Autodesk Fusion 360 part; units mm, degrees
(part 4 of 5)
  line L171 (98.6977, -61.525) -> (108.6977, -61.525)
  arc A178 (108.6977, -84.525) -> (108.6977, -81.525) centre (108.6977, -83.025) ccw
  line L172 (108.6977, -84.525) -> (98.6977, -84.525)
  arc A179 (98.6977, -81.525) -> (98.6977, -84.525) centre (98.6977, -83.025) ccw
  line L173 (98.6977, -81.525) -> (108.6977, -81.525)
  arc A180 (228.6977, -154.525) -> (228.6977, -151.525) centre (228.6977, -153.025) ccw
  line L174 (228.6977, -154.525) -> (218.6977, -154.525)
  arc A181 (218.6977, -151.525) -> (218.6977, -154.525) centre (218.6977, -153.025) ccw
  line L175 (218.6977, -151.525) -> (228.6977, -151.525)
  arc A182 (188.6977, -154.525) -> (188.6977, -151.525) centre (188.6977, -153.025) ccw
  line L176 (188.6977, -154.525) -> (178.6977, -154.525)
  arc A183 (178.6977, -151.525) -> (178.6977, -154.525) centre (178.6977, -153.025) ccw
  line L177 (178.6977, -151.525) -> (188.6977, -151.525)
  arc A184 (108.6977, -74.525) -> (108.6977, -71.525) centre (108.6977, -73.025) ccw
  line L178 (108.6977, -74.525) -> (98.6977, -74.525)
  arc A185 (98.6977, -71.525) -> (98.6977, -74.525) centre (98.6977, -73.025) ccw
  line L179 (98.6977, -71.525) -> (108.6977, -71.525)
  arc A186 (88.6977, -64.525) -> (88.6977, -61.525) centre (88.6977, -63.025) ccw
  line L180 (88.6977, -64.525) -> (78.6977, -64.525)
  arc A187 (78.6977, -61.525) -> (78.6977, -64.525) centre (78.6977, -63.025) ccw
  line L181 (78.6977, -61.525) -> (88.6977, -61.525)
  arc A188 (168.6977, -114.525) -> (168.6977, -111.525) centre (168.6977, -113.025) ccw
  line L182 (168.6977, -114.525) -> (158.6977, -114.525)
  arc A189 (158.6977, -111.525) -> (158.6977, -114.525) centre (158.6977, -113.025) ccw
  line L183 (158.6977, -111.525) -> (168.6977, -111.525)
  arc A190 (228.6977, -94.525) -> (228.6977, -91.525) centre (228.6977, -93.025) ccw
  line L184 (228.6977, -94.525) -> (218.6977, -94.525)
  arc A191 (218.6977, -91.525) -> (218.6977, -94.525) centre (218.6977, -93.025) ccw
  line L185 (218.6977, -91.525) -> (228.6977, -91.525)
  arc A192 (208.6977, -84.525) -> (208.6977, -81.525) centre (208.6977, -83.025) ccw
  line L186 (208.6977, -84.525) -> (198.6977, -84.525)
  arc A193 (198.6977, -81.525) -> (198.6977, -84.525) centre (198.6977, -83.025) ccw
  line L187 (198.6977, -81.525) -> (208.6977, -81.525)
  arc A194 (88.6977, -54.525) -> (88.6977, -51.525) centre (88.6977, -53.025) ccw
  line L188 (88.6977, -54.525) -> (78.6977, -54.525)
  arc A195 (78.6977, -51.525) -> (78.6977, -54.525) centre (78.6977, -53.025) ccw
  line L189 (78.6977, -51.525) -> (88.6977, -51.525)
  arc A196 (188.6977, -14.525) -> (188.6977, -11.525) centre (188.6977, -13.025) ccw
  line L190 (188.6977, -14.525) -> (178.6977, -14.525)
  arc A197 (178.6977, -11.525) -> (178.6977, -14.525) centre (178.6977, -13.025) ccw
  line L191 (178.6977, -11.525) -> (188.6977, -11.525)
  arc A198 (148.6977, -184.525) -> (148.6977, -181.525) centre (148.6977, -183.025) ccw
  line L192 (148.6977, -184.525) -> (138.6977, -184.525)
  arc A199 (138.6977, -181.525) -> (138.6977, -184.525) centre (138.6977, -183.025) ccw
  line L193 (138.6977, -181.525) -> (148.6977, -181.525)
  arc A200 (208.6977, -54.525) -> (208.6977, -51.525) centre (208.6977, -53.025) ccw
  line L194 (208.6977, -54.525) -> (198.6977, -54.525)
  arc A201 (198.6977, -51.525) -> (198.6977, -54.525) centre (198.6977, -53.025) ccw
  line L195 (198.6977, -51.525) -> (208.6977, -51.525)
  arc A202 (68.6977, -54.525) -> (68.6977, -51.525) centre (68.6977, -53.025) ccw
  line L196 (68.6977, -54.525) -> (58.6977, -54.525)
  arc A203 (58.6977, -51.525) -> (58.6977, -54.525) centre (58.6977, -53.025) ccw
  line L197 (58.6977, -51.525) -> (68.6977, -51.525)
  arc A204 (208.6977, -64.525) -> (208.6977, -61.525) centre (208.6977, -63.025) ccw
  line L198 (208.6977, -64.525) -> (198.6977, -64.525)
  arc A205 (198.6977, -61.525) -> (198.6977, -64.525) centre (198.6977, -63.025) ccw
  line L199 (198.6977, -61.525) -> (208.6977, -61.525)
  arc A206 (208.6977, -174.525) -> (208.6977, -171.525) centre (208.6977, -173.025) ccw
  line L200 (208.6977, -174.525) -> (198.6977, -174.525)
  arc A207 (198.6977, -171.525) -> (198.6977, -174.525) centre (198.6977, -173.025) ccw
  line L201 (198.6977, -171.525) -> (208.6977, -171.525)
  arc A208 (168.6977, -144.525) -> (168.6977, -141.525) centre (168.6977, -143.025) ccw
  line L202 (168.6977, -144.525) -> (158.6977, -144.525)
  arc A209 (158.6977, -141.525) -> (158.6977, -144.525) centre (158.6977, -143.025) ccw
  line L203 (158.6977, -141.525) -> (168.6977, -141.525)
  arc A210 (68.6977, -64.525) -> (68.6977, -61.525) centre (68.6977, -63.025) ccw
  line L204 (68.6977, -64.525) -> (58.6977, -64.525)
  arc A211 (58.6977, -61.525) -> (58.6977, -64.525) centre (58.6977, -63.025) ccw
  line L205 (58.6977, -61.525) -> (68.6977, -61.525)
  arc A212 (248.6977, -124.525) -> (248.6977, -121.525) centre (248.6977, -123.025) ccw
  line L206 (248.6977, -124.525) -> (238.6977, -124.525)
  arc A213 (238.6977, -121.525) -> (238.6977, -124.525) centre (238.6977, -123.025) ccw
  line L207 (238.6977, -121.525) -> (248.6977, -121.525)
  arc A214 (228.6977, -124.525) -> (228.6977, -121.525) centre (228.6977, -123.025) ccw
  line L208 (228.6977, -124.525) -> (218.6977, -124.525)
  arc A215 (218.6977, -121.525) -> (218.6977, -124.525) centre (218.6977, -123.025) ccw
  line L209 (218.6977, -121.525) -> (228.6977, -121.525)
  arc A216 (208.6977, -144.525) -> (208.6977, -141.525) centre (208.6977, -143.025) ccw
  line L210 (208.6977, -144.525) -> (198.6977, -144.525)
  arc A217 (198.6977, -141.525) -> (198.6977, -144.525) centre (198.6977, -143.025) ccw
  line L211 (198.6977, -141.525) -> (208.6977, -141.525)
  arc A218 (148.6977, -134.525) -> (148.6977, -131.525) centre (148.6977, -133.025) ccw
  line L212 (148.6977, -134.525) -> (138.6977, -134.525)
  arc A219 (138.6977, -131.525) -> (138.6977, -134.525) centre (138.6977, -133.025) ccw
  line L213 (138.6977, -131.525) -> (148.6977, -131.525)
  arc A220 (188.6977, -64.525) -> (188.6977, -61.525) centre (188.6977, -63.025) ccw
  line L214 (188.6977, -64.525) -> (178.6977, -64.525)
  arc A221 (178.6977, -61.525) -> (178.6977, -64.525) centre (178.6977, -63.025) ccw
  line L215 (178.6977, -61.525) -> (188.6977, -61.525)
  arc A222 (168.6977, -174.525) -> (168.6977, -171.525) centre (168.6977, -173.025) ccw
  line L216 (168.6977, -174.525) -> (158.6977, -174.525)
  arc A223 (158.6977, -171.525) -> (158.6977, -174.525) centre (158.6977, -173.025) ccw
  line L217 (158.6977, -171.525) -> (168.6977, -171.525)
  arc A224 (228.6977, -114.525) -> (228.6977, -111.525) centre (228.6977, -113.025) ccw
  line L218 (228.6977, -114.525) -> (218.6977, -114.525)
  arc A225 (218.6977, -111.525) -> (218.6977, -114.525) centre (218.6977, -113.025) ccw
  line L219 (218.6977, -111.525) -> (228.6977, -111.525)
  arc A226 (128.6977, -94.525) -> (128.6977, -91.525) centre (128.6977, -93.025) ccw
  line L220 (128.6977, -94.525) -> (118.6977, -94.525)
  arc A227 (118.6977, -91.525) -> (118.6977, -94.525) centre (118.6977, -93.025) ccw
  line L221 (118.6977, -91.525) -> (128.6977, -91.525)
  arc A228 (168.6977, 5.475) -> (168.6977, 8.475) centre (168.6977, 6.975) ccw
  line L222 (168.6977, 5.475) -> (158.6977, 5.475)
  arc A229 (158.6977, 8.475) -> (158.6977, 5.475) centre (158.6977, 6.975) ccw
  line L223 (158.6977, 8.475) -> (168.6977, 8.475)
  arc A230 (188.6977, -74.525) -> (188.6977, -71.525) centre (188.6977, -73.025) ccw
  line L224 (188.6977, -74.525) -> (178.6977, -74.525)
  arc A231 (178.6977, -71.525) -> (178.6977, -74.525) centre (178.6977, -73.025) ccw
  line L225 (178.6977, -71.525) -> (188.6977, -71.525)
  arc A232 (108.6977, -114.525) -> (108.6977, -111.525) centre (108.6977, -113.025) ccw
  line L226 (108.6977, -114.525) -> (98.6977, -114.525)
  arc A233 (98.6977, -111.525) -> (98.6977, -114.525) centre (98.6977, -113.025) ccw
  line L227 (98.6977, -111.525) -> (108.6977, -111.525)
  arc A234 (208.6977, -104.525) -> (208.6977, -101.525) centre (208.6977, -103.025) ccw
  line L228 (208.6977, -104.525) -> (198.6977, -104.525)
  arc A235 (198.6977, -101.525) -> (198.6977, -104.525) centre (198.6977, -103.025) ccw
  line L229 (198.6977, -101.525) -> (208.6977, -101.525)
  arc A236 (208.6977, -154.525) -> (208.6977, -151.525) centre (208.6977, -153.025) ccw
  line L230 (208.6977, -154.525) -> (198.6977, -154.525)
  arc A237 (198.6977, -151.525) -> (198.6977, -154.525) centre (198.6977, -153.025) ccw
  line L231 (198.6977, -151.525) -> (208.6977, -151.525)
  arc A238 (168.6977, -104.525) -> (168.6977, -101.525) centre (168.6977, -103.025) ccw
  line L232 (168.6977, -104.525) -> (158.6977, -104.525)
  arc A239 (158.6977, -101.525) -> (158.6977, -104.525) centre (158.6977, -103.025) ccw
  line L233 (158.6977, -101.525) -> (168.6977, -101.525)
  arc A240 (188.6977, -174.525) -> (188.6977, -171.525) centre (188.6977, -173.025) ccw
  line L234 (188.6977, -174.525) -> (178.6977, -174.525)
  arc A241 (178.6977, -171.525) -> (178.6977, -174.525) centre (178.6977, -173.025) ccw
  line L235 (178.6977, -171.525) -> (188.6977, -171.525)
  arc A242 (248.6977, -64.525) -> (248.6977, -61.525) centre (248.6977, -63.025) ccw
  line L236 (248.6977, -64.525) -> (238.6977, -64.525)
  arc A243 (238.6977, -61.525) -> (238.6977, -64.525) centre (238.6977, -63.025) ccw
  line L237 (238.6977, -61.525) -> (248.6977, -61.525)
  arc A244 (128.6977, -84.525) -> (128.6977, -81.525) centre (128.6977, -83.025) ccw
  line L238 (128.6977, -84.525) -> (118.6977, -84.525)
  arc A245 (118.6977, -81.525) -> (118.6977, -84.525) centre (118.6977, -83.025) ccw
  line L239 (118.6977, -81.525) -> (128.6977, -81.525)
  arc A246 (88.6977, -114.525) -> (88.6977, -111.525) centre (88.6977, -113.025) ccw
  line L240 (88.6977, -114.525) -> (78.6977, -114.525)
  arc A247 (78.6977, -111.525) -> (78.6977, -114.525) centre (78.6977, -113.025) ccw
  line L241 (78.6977, -111.525) -> (88.6977, -111.525)
  line L242 (46.3999, -83.0262) -> (46.3999, -63.0262)
  line L243 (46.3999, -63.0262) -> (53.3999, -63.0262)
  line L244 (53.3999, -63.0262) -> (53.3999, -83.0262)
  line L245 (53.3999, -83.0262) -> (46.3999, -83.0262)
  arc A248 (230.0109, -143.75) -> (228.6869, -141.525) centre (230, -142.25) ccw
  arc A249 (228.6977, -144.525) -> (230.0109, -143.75) centre (228.6977, -143.025) ccw
  line L246 (228.6977, -144.525) -> (218.6977, -144.525)
  arc A250 (218.6977, -141.525) -> (218.6977, -144.525) centre (218.6977, -143.025) ccw
  line L247 (218.6977, -141.525) -> (228.6869, -141.525)
  arc A251 (168.6977, -94.525) -> (168.6977, -91.525) centre (168.6977, -93.025) ccw
  line L248 (168.6977, -94.525) -> (158.6977, -94.525)
  arc A252 (158.6977, -91.525) -> (158.6977, -94.525) centre (158.6977, -93.025) ccw
  line L249 (158.6977, -91.525) -> (168.6977, -91.525)
  arc A253 (248.6977, -114.525) -> (248.6977, -111.525) centre (248.6977, -113.025) ccw
  line L250 (248.6977, -114.525) -> (238.6977, -114.525)
  arc A254 (238.6977, -111.525) -> (238.6977, -114.525) centre (238.6977, -113.025) ccw
  line L251 (238.6977, -111.525) -> (248.6977, -111.525)
  arc A255 (168.6977, -54.525) -> (168.6977, -51.525) centre (168.6977, -53.025) ccw
  line L252 (168.6977, -54.525) -> (158.6977, -54.525)
  arc A256 (158.6977, -51.525) -> (158.6977, -54.525) centre (158.6977, -53.025) ccw
  line L253 (158.6977, -51.525) -> (168.6977, -51.525)
  arc A257 (168.6977, -74.525) -> (168.6977, -71.525) centre (168.6977, -73.025) ccw
  line L254 (168.6977, -74.525) -> (158.6977, -74.525)
  arc A258 (158.6977, -71.525) -> (158.6977, -74.525) centre (158.6977, -73.025) ccw
  line L255 (158.6977, -71.525) -> (168.6977, -71.525)
  arc A259 (248.6977, -104.525) -> (248.6977, -101.525) centre (248.6977, -103.025) ccw
  line L256 (248.6977, -104.525) -> (238.6977, -104.525)
  arc A260 (238.6977, -101.525) -> (238.6977, -104.525) centre (238.6977, -103.025) ccw
  line L257 (238.6977, -101.525) -> (248.6977, -101.525)
  arc A261 (228.6977, -164.525) -> (228.6977, -161.525) centre (228.6977, -163.025) ccw
  line L258 (228.6977, -164.525) -> (218.6977, -164.525)
  arc A262 (218.6977, -161.525) -> (218.6977, -164.525) centre (218.6977, -163.025) ccw
  line L259 (218.6977, -161.525) -> (228.6977, -161.525)
  arc A263 (208.6977, -164.525) -> (208.6977, -161.525) centre (208.6977, -163.025) ccw
  line L260 (208.6977, -164.525) -> (198.6977, -164.525)
  arc A264 (198.6977, -161.525) -> (198.6977, -164.525) centre (198.6977, -163.025) ccw
  line L261 (198.6977, -161.525) -> (208.6977, -161.525)
  arc A265 (188.6977, -144.525) -> (188.6977, -141.525) centre (188.6977, -143.025) ccw
  line L262 (188.6977, -144.525) -> (178.6977, -144.525)
  arc A266 (178.6977, -141.525) -> (178.6977, -144.525) centre (178.6977, -143.025) ccw
  line L263 (178.6977, -141.525) -> (188.6977, -141.525)
  arc A267 (188.6977, 35.475) -> (188.6977, 38.475) centre (188.6977, 36.975) ccw
  line L264 (188.6977, 35.475) -> (178.6977, 35.475)
  arc A268 (178.6977, 38.475) -> (178.6977, 35.475) centre (178.6977, 36.975) ccw
  line L265 (178.6977, 38.475) -> (188.6977, 38.475)
  arc A269 (188.6977, -54.525) -> (188.6977, -51.525) centre (188.6977, -53.025) ccw
  line L266 (188.6977, -54.525) -> (178.6977, -54.525)
  arc A270 (178.6977, -51.525) -> (178.6977, -54.525) centre (178.6977, -53.025) ccw
  line L267 (178.6977, -51.525) -> (188.6977, -51.525)
  arc A271 (128.6977, -134.525) -> (128.6977, -131.525) centre (128.6977, -133.025) ccw
  line L268 (128.6977, -134.525) -> (118.6977, -134.525)
  arc A272 (118.6977, -131.525) -> (118.6977, -134.525) centre (118.6977, -133.025) ccw
  line L269 (118.6977, -131.525) -> (128.6977, -131.525)
  arc A273 (88.6977, -84.525) -> (88.6977, -81.525) centre (88.6977, -83.025) ccw
  line L270 (88.6977, -84.525) -> (78.6977, -84.525)
  arc A274 (78.6977, -81.525) -> (78.6977, -84.525) centre (78.6977, -83.025) ccw
  line L271 (78.6977, -81.525) -> (88.6977, -81.525)
  arc A275 (188.6977, -84.525) -> (188.6977, -81.525) centre (188.6977, -83.025) ccw
  line L272 (188.6977, -84.525) -> (178.6977, -84.525)
  arc A276 (178.6977, -81.525) -> (178.6977, -84.525) centre (178.6977, -83.025) ccw
  line L273 (178.6977, -81.525) -> (188.6977, -81.525)
  arc A277 (188.6977, 15.475) -> (188.6977, 18.475) centre (188.6977, 16.975) ccw
  line L274 (188.6977, 15.475) -> (178.6977, 15.475)
  arc A278 (178.6977, 18.475) -> (178.6977, 15.475) centre (178.6977, 16.975) ccw
  line L275 (178.6977, 18.475) -> (188.6977, 18.475)
  arc A279 (128.6977, -114.525) -> (128.6977, -111.525) centre (128.6977, -113.025) ccw
  line L276 (128.6977, -114.525) -> (118.6977, -114.525)
  arc A280 (118.6977, -111.525) -> (118.6977, -114.525) centre (118.6977, -113.025) ccw
  line L277 (118.6977, -111.525) -> (128.6977, -111.525)
  arc A281 (248.6977, -84.525) -> (248.6977, -81.525) centre (248.6977, -83.025) ccw
  line L278 (248.6977, -84.525) -> (238.6977, -84.525)
  arc A282 (238.6977, -81.525) -> (238.6977, -84.525) centre (238.6977, -83.025) ccw
  line L279 (238.6977, -81.525) -> (248.6977, -81.525)
  arc A283 (88.6977, -104.525) -> (88.6977, -101.525) centre (88.6977, -103.025) ccw
  line L280 (88.6977, -104.525) -> (78.6977, -104.525)
  arc A284 (78.6977, -101.525) -> (78.6977, -104.525) centre (78.6977, -103.025) ccw
  line L281 (78.6977, -101.525) -> (88.6977, -101.525)
  arc A285 (128.6977, -154.525) -> (128.6977, -151.525) centre (128.6977, -153.025) ccw
  line L282 (128.6977, -154.525) -> (118.6977, -154.525)
  arc A286 (118.6977, -151.525) -> (118.6977, -154.525) centre (118.6977, -153.025) ccw
  line L283 (118.6977, -151.525) -> (128.6977, -151.525)
  arc A287 (228.6977, -104.525) -> (228.6977, -101.525) centre (228.6977, -103.025) ccw
  line L284 (228.6977, -104.525) -> (218.6977, -104.525)
  arc A288 (218.6977, -101.525) -> (218.6977, -104.525) centre (218.6977, -103.025) ccw
  line L285 (218.6977, -101.525) -> (228.6977, -101.525)
  arc A289 (188.6977, -134.525) -> (188.6977, -131.525) centre (188.6977, -133.025) ccw
  line L286 (188.6977, -134.525) -> (178.6977, -134.525)
  arc A290 (178.6977, -131.525) -> (178.6977, -134.525) centre (178.6977, -133.025) ccw
  line L287 (178.6977, -131.525) -> (188.6977, -131.525)
  arc A291 (228.6977, -74.525) -> (228.6977, -71.525) centre (228.6977, -73.025) ccw
  line L288 (228.6977, -74.525) -> (218.6977, -74.525)
  arc A292 (218.6977, -71.525) -> (218.6977, -74.525) centre (218.6977, -73.025) ccw
  line L289 (218.6977, -71.525) -> (228.6977, -71.525)
  arc A293 (188.6977, -104.525) -> (188.6977, -101.525) centre (188.6977, -103.025) ccw
  line L290 (188.6977, -104.525) -> (178.6977, -104.525)
  arc A294 (178.6977, -101.525) -> (178.6977, -104.525) centre (178.6977, -103.025) ccw
  line L291 (178.6977, -101.525) -> (188.6977, -101.525)
  arc A295 (208.6977, -124.525) -> (208.6977, -121.525) centre (208.6977, -123.025) ccw
  line L292 (208.6977, -124.525) -> (198.6977, -124.525)
  arc A296 (198.6977, -121.525) -> (198.6977, -124.525) centre (198.6977, -123.025) ccw
  line L293 (198.6977, -121.525) -> (208.6977, -121.525)
  arc A297 (68.6977, -84.525) -> (68.6977, -81.525) centre (68.6977, -83.025) ccw
  line L294 (68.6977, -84.525) -> (58.6977, -84.525)
  arc A298 (58.6977, -81.525) -> (58.6977, -84.525) centre (58.6977, -83.025) ccw
  line L295 (58.6977, -81.525) -> (68.6977, -81.525)
  arc A299 (148.6977, -54.525) -> (148.6977, -51.525) centre (148.6977, -53.025) ccw
  line L296 (148.6977, -54.525) -> (138.6977, -54.525)
  arc A300 (138.6977, -51.525) -> (138.6977, -54.525) centre (138.6977, -53.025) ccw
  line L297 (138.6977, -51.525) -> (148.6977, -51.525)
  arc A301 (248.6977, -94.525) -> (248.6977, -91.525) centre (248.6977, -93.025) ccw
  line L298 (248.6977, -94.525) -> (238.6977, -94.525)
  arc A302 (238.6977, -91.525) -> (238.6977, -94.525) centre (238.6977, -93.025) ccw
  line L299 (238.6977, -91.525) -> (248.6977, -91.525)
  arc A303 (208.6977, -184.525) -> (208.6977, -181.525) centre (208.6977, -183.025) ccw
  line L300 (208.6977, -184.525) -> (198.6977, -184.525)
  arc A304 (198.6977, -181.525) -> (198.6977, -184.525) centre (198.6977, -183.025) ccw
  line L301 (198.6977, -181.525) -> (208.6977, -181.525)
  arc A305 (108.6977, -94.525) -> (108.6977, -91.525) centre (108.6977, -93.025) ccw
  line L302 (108.6977, -94.525) -> (98.6977, -94.525)
  arc A306 (98.6977, -91.525) -> (98.6977, -94.525) centre (98.6977, -93.025) ccw
  line L303 (98.6977, -91.525) -> (108.6977, -91.525)
  arc A307 (128.6977, -14.525) -> (128.6977, -11.525) centre (128.6977, -13.025) ccw
  line L304 (128.6977, -14.525) -> (118.6977, -14.525)
  arc A308 (118.6977, -11.525) -> (118.6977, -14.525) centre (118.6977, -13.025) ccw
  line L305 (118.6977, -11.525) -> (128.6977, -11.525)
  arc A309 (188.6977, -94.525) -> (188.6977, -91.525) centre (188.6977, -93.025) ccw
  line L306 (188.6977, -94.525) -> (178.6977, -94.525)
  arc A310 (178.6977, -91.525) -> (178.6977, -94.525) centre (178.6977, -93.025) ccw
  line L307 (178.6977, -91.525) -> (188.6977, -91.525)
  arc A311 (168.6977, -134.525) -> (168.6977, -131.525) centre (168.6977, -133.025) ccw
  line L308 (168.6977, -134.525) -> (158.6977, -134.525)
  arc A312 (158.6977, -131.525) -> (158.6977, -134.525) centre (158.6977, -133.025) ccw
  line L309 (158.6977, -131.525) -> (168.6977, -131.525)
  arc A313 (128.6977, -144.525) -> (128.6977, -141.525) centre (128.6977, -143.025) ccw
  line L310 (128.6977, -144.525) -> (118.6977, -144.525)
  arc A314 (118.6977, -141.525) -> (118.6977, -144.525) centre (118.6977, -143.025) ccw
  line L311 (118.6977, -141.525) -> (128.6977, -141.525)
  arc A315 (88.6977, -74.525) -> (88.6977, -71.525) centre (88.6977, -73.025) ccw
  line L312 (88.6977, -74.525) -> (78.6977, -74.525)
  arc A316 (78.6977, -71.525) -> (78.6977, -74.525) centre (78.6977, -73.025) ccw
  line L313 (78.6977, -71.525) -> (88.6977, -71.525)
  arc A317 (148.6977, -84.525) -> (148.6977, -81.525) centre (148.6977, -83.025) ccw
  line L314 (148.6977, -84.525) -> (138.6977, -84.525)
  arc A318 (138.6977, -81.525) -> (138.6977, -84.525) centre (138.6977, -83.025) ccw
  line L315 (138.6977, -81.525) -> (148.6977, -81.525)
  arc A319 (108.6977, -104.525) -> (108.6977, -101.525) centre (108.6977, -103.025) ccw
  line L316 (108.6977, -104.525) -> (98.6977, -104.525)
  arc A320 (98.6977, -101.525) -> (98.6977, -104.525) centre (98.6977, -103.025) ccw
  line L317 (98.6977, -101.525) -> (108.6977, -101.525)
  arc A321 (168.6977, -84.525) -> (168.6977, -81.525) centre (168.6977, -83.025) ccw
  line L318 (168.6977, -84.525) -> (158.6977, -84.525)
  arc A322 (158.6977, -81.525) -> (158.6977, -84.525) centre (158.6977, -83.025) ccw
  line L319 (158.6977, -81.525) -> (168.6977, -81.525)
  arc A323 (228.6977, -64.525) -> (228.6977, -61.525) centre (228.6977, -63.025) ccw
  line L320 (228.6977, -64.525) -> (218.6977, -64.525)
  arc A324 (218.6977, -61.525) -> (218.6977, -64.525) centre (218.6977, -63.025) ccw
  line L321 (218.6977, -61.525) -> (228.6977, -61.525)
  arc A325 (228.6977, -84.525) -> (228.6977, -81.525) centre (228.6977, -83.025) ccw
  line L322 (228.6977, -84.525) -> (218.6977, -84.525)
  arc A326 (218.6977, -81.525) -> (218.6977, -84.525) centre (218.6977, -83.025) ccw
  line L323 (218.6977, -81.525) -> (228.6977, -81.525)
  arc A327 (148.6977, -114.525) -> (148.6977, -111.525) centre (148.6977, -113.025) ccw
  line L324 (148.6977, -114.525) -> (138.6977, -114.525)
  arc A328 (138.6977, -111.525) -> (138.6977, -114.525) centre (138.6977, -113.025) ccw
  line L325 (138.6977, -111.525) -> (148.6977, -111.525)
  arc A329 (168.6977, -154.525) -> (168.6977, -151.525) centre (168.6977, -153.025) ccw
  line L326 (168.6977, -154.525) -> (158.6977, -154.525)
  arc A330 (158.6977, -151.525) -> (158.6977, -154.525) centre (158.6977, -153.025) ccw
  line L327 (158.6977, -151.525) -> (168.6977, -151.525)
  arc A331 (68.6977, -74.525) -> (68.6977, -71.525) centre (68.6977, -73.025) ccw
  line L328 (68.6977, -74.525) -> (58.6977, -74.525)
  arc A332 (58.6977, -71.525) -> (58.6977, -74.525) centre (58.6977, -73.025) ccw
  line L329 (58.6977, -71.525) -> (68.6977, -71.525)
  arc A333 (128.6977, -64.525) -> (128.6977, -61.525) centre (128.6977, -63.025) ccw
  line L330 (128.6977, -64.525) -> (118.6977, -64.525)
  arc A334 (118.6977, -61.525) -> (118.6977, -64.525) centre (118.6977, -63.025) ccw
  line L331 (118.6977, -61.525) -> (128.6977, -61.525)
  arc A335 (248.6977, -134.525) -> (248.6977, -131.525) centre (248.6977, -133.025) ccw
  line L332 (248.6977, -134.525) -> (238.6977, -134.525)
  arc A336 (238.6977, -131.525) -> (238.6977, -134.525) centre (238.6977, -133.025) ccw
  line L333 (238.6977, -131.525) -> (248.6977, -131.525)
  arc A337 (128.6977, -104.525) -> (128.6977, -101.525) centre (128.6977, -103.025) ccw
  line L334 (128.6977, -104.525) -> (118.6977, -104.525)
  arc A338 (118.6977, -101.525) -> (118.6977, -104.525) centre (118.6977, -103.025) ccw
  line L335 (118.6977, -101.525) -> (128.6977, -101.525)
  arc A339 (208.6977, -4.525) -> (208.6977, -1.525) centre (208.6977, -3.025) ccw
  line L336 (208.6977, -4.525) -> (198.6977, -4.525)
  arc A340 (198.6977, -1.525) -> (198.6977, -4.525) centre (198.6977, -3.025) ccw
  line L337 (198.6977, -1.525) -> (208.6977, -1.525)
  arc A341 (208.6977, -134.525) -> (208.6977, -131.525) centre (208.6977, -133.025) ccw
  line L338 (208.6977, -134.525) -> (198.6977, -134.525)
  arc A342 (198.6977, -131.525) -> (198.6977, -134.525) centre (198.6977, -133.025) ccw
  line L339 (198.6977, -131.525) -> (208.6977, -131.525)
  arc A343 (128.6977, -124.525) -> (128.6977, -121.525) centre (128.6977, -123.025) ccw
  line L340 (128.6977, -124.525) -> (118.6977, -124.525)
  arc A344 (118.6977, -121.525) -> (118.6977, -124.525) centre (118.6977, -123.025) ccw
  line L341 (118.6977, -121.525) -> (128.6977, -121.525)
  arc A345 (128.6977, -54.525) -> (128.6977, -51.525) centre (128.6977, -53.025) ccw
  line L342 (128.6977, -54.525) -> (118.6977, -54.525)
  arc A346 (118.6977, -51.525) -> (118.6977, -54.525) centre (118.6977, -53.025) ccw
  line L343 (118.6977, -51.525) -> (128.6977, -51.525)
  arc A347 (208.6977, -14.525) -> (208.6977, -11.525) centre (208.6977, -13.025) ccw
  line L344 (208.6977, -14.525) -> (198.6977, -14.525)
  arc A348 (198.6977, -11.525) -> (198.6977, -14.525) centre (198.6977, -13.025) ccw
  line L345 (198.6977, -11.525) -> (208.6977, -11.525)
  arc A349 (108.6977, -134.525) -> (108.6977, -131.525) centre (108.6977, -133.025) ccw
  line L346 (108.6977, -134.525) -> (98.6977, -134.525)
  arc A350 (98.6977, -131.525) -> (98.6977, -134.525) centre (98.6977, -133.025) ccw
  line L347 (98.6977, -131.525) -> (108.6977, -131.525)
  arc A351 (88.6977, -94.525) -> (88.6977, -91.525) centre (88.6977, -93.025) ccw
  line L348 (88.6977, -94.525) -> (78.6977, -94.525)
  arc A352 (78.6977, -91.525) -> (78.6977, -94.525) centre (78.6977, -93.025) ccw
  line L349 (78.6977, -91.525) -> (88.6977, -91.525)
  arc A353 (148.6977, -174.525) -> (148.6977, -171.525) centre (148.6977, -173.025) ccw
  line L350 (148.6977, -174.525) -> (138.6977, -174.525)
  arc A354 (138.6977, -171.525) -> (138.6977, -174.525) centre (138.6977, -173.025) ccw
  line L351 (138.6977, -171.525) -> (148.6977, -171.525)
  arc A355 (108.6977, -124.525) -> (108.6977, -121.525) centre (108.6977, -123.025) ccw
  line L352 (108.6977, -124.525) -> (98.6977, -124.525)
  arc A356 (98.6977, -121.525) -> (98.6977, -124.525) centre (98.6977, -123.025) ccw
  line L353 (98.6977, -121.525) -> (108.6977, -121.525)
component "Electronics Plate" placed x (1, 0, 0) y (0, 1, 0) z (0, 0, 1) at (0, 0, 0)

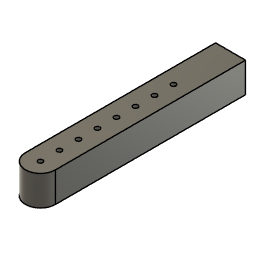
design "Camera arm 2"
Autodesk Fusion 360 part; units mm, degrees
sketch "Sketch1" plane through (0, 0, 0) normal (0, 1, 0) x (1, 0, 0)
  line L0 (20, 0) -> (20, -127)
  line L1 (0, -127) -> (0, 0)
  arc A0 (0, -127) -> (20, -127) centre (10, -127) ccw
  line L2 (0, 0) -> (20, 0)
  circle A1 centre (10, -127) radius 1.6
  dimension "d1" = 20
  dimension "d2" = 127
  dimension "d3" = 3.2
  constraint vertical L0
  constraint vertical L1
  constraint coincident L1.end L2.start
  constraint perpendicular L0 L2
  constraint concentric A0 A1
  measures "d1" distance of L1.end L0.start
  measures "d2" distance of L1.end L1.start
  measures "d3" diameter of A1
extrude "Extrude1" add sketch "Sketch1" along normal blind 20
sketch "Sketch2" plane through (0, 0, 0) normal (0, 0, -1) x (-1, 0, 0)
  line L0 (-20, 0) -> (0, 0)
  line L1 (0, 0) -> (0, 20)
  line L2 (0, 20) -> (-20, 20)
  line L3 (-20, 20) -> (-20, 0)
  line L4 (-20, 20) -> (0, 20)
  line L5 (0, 20) -> (0, 0)
  line L6 (0, 0) -> (-20, 0)
  line L7 (-20, 0) -> (-20, 20)
  circle A0 centre (-16, 16) radius 1
  circle A1 centre (-4, 16) radius 1
  circle A2 centre (-16, 4) radius 1
  circle A3 centre (-4, 4) radius 1
  dimension "d6" = 2
  dimension "d7" = 2
  dimension "d8" = 2
  dimension "d9" = 2
  dimension "d16" = 4
  dimension "d17" = 4
  dimension "d18" = 4
  dimension "d19" = 4
  dimension "d20" = 4
  dimension "d21" = 4
  dimension "d22" = 4
  dimension "d23" = 4
  constraint horizontal L4
  constraint vertical L5
  constraint horizontal L6
  constraint vertical L7
  constraint coincident L0.end L1.start
  constraint coincident L2.end L3.start
  measures "d6" diameter of A0
  measures "d7" diameter of A1
  measures "d8" diameter of A2
  measures "d9" diameter of A3
  measures "d16" distance of L4 A0.centre
  measures "d17" distance of L7 A0.centre
  measures "d18" distance of L4 A1.centre
  measures "d19" distance of L5 A1.centre
  measures "d20" distance of L5 A3.centre
  measures "d21" distance of L6 A3.centre
  measures "d22" distance of L7 A2.centre
  measures "d23" distance of L6 A2.centre
extrude "Extrude2" cut sketch "Sketch2" against normal blind 40 contours A0 | A1 | A2 | A3
sketch "Sketch3" plane through (0, 20, 0) normal (0, 1, 0) x (-1, 0, 0)
  circle A0 centre (-10, 127) radius 1.6
  arc A1 (0, 127) -> (-20, 127) centre (-10, 127) ccw
  line L0 (-20, 127) -> (-20, 0)
  line L1 (-20, 0) -> (0, 0)
  line L2 (0, 0) -> (0, 127)
  circle A2 centre (-10, 114.3) radius 1.6
  circle A3 centre (-10, 101.6) radius 1.6
  circle A4 centre (-10, 88.9) radius 1.6
  circle A5 centre (-10, 76.2) radius 1.6
  circle A6 centre (-10, 63.5) radius 1.6
  circle A7 centre (-10, 50.8) radius 1.6
  circle A8 centre (-10, 38.1) radius 1.6
  dimension "d24" = 3.2
  dimension "d25" = 12.7
  dimension "d28" = 0
  dimension "d29" = -12.7
  measures "d24" diameter of A2
  measures "d25" distance of A0.centre A2.centre
extrude "Extrude3" cut sketch "Sketch3" against normal blind 170 contours A2 | A3 | A4 | A5 | A6 | A7 | A8

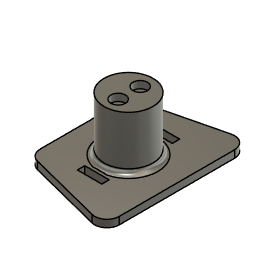
design "Lock"
Autodesk Fusion 360 part; units mm, degrees
sketch "Sketch1" plane through (0, 0, 0) normal (0, 1, 0) x (1, 0, 0)
  line L0 (46.0121, 0.2) -> (46.0121, -59.8)
  line L1 (6.0121, -29.5532) -> (6.0121, -9.5532)
  line L2 (6.0121, -29.5532) -> (6.0121, -49.5532)
  line L3 (6.0121, -9.5532) -> (46.0121, 0.2)
  line L4 (6.0121, -49.5532) -> (46.0121, -59.8)
  line L5 (31.0121, -13.6532) -> (21.0121, -13.6532)
  line L6 (21.0121, -13.6532) -> (21.0121, -16.6532)
  line L7 (21.0121, -16.6532) -> (31.0121, -16.6532)
  line L8 (31.0121, -16.6532) -> (31.0121, -13.6532)
  line L9 (31.0121, -42.4532) -> (21.0121, -42.4532)
  line L10 (21.0121, -42.4532) -> (21.0121, -45.4532)
  line L11 (21.0121, -45.4532) -> (31.0121, -45.4532)
  line L12 (31.0121, -45.4532) -> (31.0121, -42.4532)
  point P0 (26.0121, -15.0532)
  point P1 (25.8317, -44.4989)
  dimension "d1" = 60
  dimension "d6" = 20
  dimension "d7" = 20
  dimension "d9" = 40
  dimension "d10" = 40
  dimension "d11" = 20
  dimension "d12" = 14.5
  dimension "d13" = 10
  dimension "d14" = 3
  dimension "d15" = 10
  dimension "d16" = 3
  dimension "d19" = 12.9
  dimension "d20" = 12.9
  dimension "d21" = 25.8
  dimension "d22" = 15
  dimension "d23" = 15
  constraint parallel L0 L1
  constraint parallel L1 L2
  constraint horizontal L5
  constraint perpendicular L5 L6
  constraint parallel L5 L7
  constraint parallel L6 L8
  constraint horizontal L9
  constraint perpendicular L9 L10
  constraint parallel L9 L11
  constraint parallel L10 L12
  measures "d1" distance of L0.start L0.end
  measures "d6" distance of L1.start L1.end
  measures "d7" distance of L1.start L2.end
  measures "d9" distance of L0 L2
  measures "d10" distance of L1.end L2.end
  measures "d11" distance of L0 P0
  measures "d12" vertical distance of L1.start P0
  measures "d13" distance of L6.end L7.end
  measures "d14" distance of L5.end L6.end
  measures "d15" distance of L10.end L11.end
  measures "d16" distance of L9.end L10.end
  measures "d19" distance of L1.start L9
  measures "d20" vertical distance of L1.start L6.end
  measures "d21" distance of L7 L9
  measures "d22" distance of L2 L10
  measures "d23" distance of L1 L6
extrude "Extrude1" add sketch "Sketch1" along normal blind 3
sketch "Sketch2" plane through (0, 3, 0) normal (0, 1, 0) x (-1, 0, 0)
  line L0 (-31.0121, 42.4532) -> (-31.0121, 45.4532)
  line L1 (-31.0121, 45.4532) -> (-21.0121, 45.4532)
  line L2 (-21.0121, 45.4532) -> (-21.0121, 42.4532)
  line L3 (-21.0121, 42.4532) -> (-31.0121, 42.4532)
  line L4 (-31.0121, 13.6532) -> (-31.0121, 16.6532)
  line L5 (-31.0121, 16.6532) -> (-21.0121, 16.6532)
  line L6 (-21.0121, 16.6532) -> (-21.0121, 13.6532)
  line L7 (-21.0121, 13.6532) -> (-31.0121, 13.6532)
  line L8 (-6.0121, 9.5532) -> (-6.0121, 49.5532)
  line L9 (-6.0121, 49.5532) -> (-46.0121, 59.8)
  line L10 (-46.0121, 59.8) -> (-46.0121, -0.2)
  line L11 (-46.0121, -0.2) -> (-6.0121, 9.5532)
  circle A0 centre (-26.0121, 29.5532) radius 10
  point P0 (-26.0121, 29.5532)
  dimension "d38" = 12.9
  dimension "d39" = 12.9
  dimension "d42" = 20
  constraint coincident P0 A0.centre
  measures "d38" distance of L3 P0
  measures "d39" distance of L5 P0
  measures "d42" diameter of A0
extrude "Extrude2" add sketch "Sketch2" along normal blind 22 contours A0
sketch "Sketch3" plane through (0, 25, 0) normal (0, 1, 0) x (-1, 0, 0)
  line L0 (-28.0121, 38.7532) -> (-24.0121, 38.7532)
  line L1 (-24.0121, 38.7532) -> (-24.0121, 20.7532)
  line L2 (-24.0121, 20.7532) -> (-28.0121, 20.7532)
  line L3 (-28.0121, 20.7532) -> (-28.0121, 38.7532)
  line L4 (-28.0121, 38.7532) -> (-24.0121, 20.7532) construction
  line L5 (-24.0121, 38.7532) -> (-28.0121, 20.7532) construction
  circle A0 centre (-26.0121, 29.5532) radius 10
  point P0 (-26.0121, 29.7532)
  dimension "d28" = 18
  constraint horizontal L0
  constraint perpendicular L0 L1
  constraint parallel L0 L2
  constraint parallel L1 L3
  constraint coincident L4 P0
  constraint coincident L5 P0
  measures "d28" distance of L0.end L1.end
fillet "Fillet4" radius 2 1 edges at (35.3354, 3, 33.1694)
fillet "Fillet3" radius 5 4 edges at (6.0121, 1.5, 9.5532) (6.0121, 1.5, 49.5532) (46.0121, 1.5, 59.8) (46.0121, 1.5, -0.2)
sketch "Sketch5" plane through (0, 25, 0) normal (0, 1, 0) x (-1, 0, 0)
  circle A0 centre (-26.0121, 29.5532) radius 10
  circle A1 centre (-26.282, 34.0532) radius 2.975
  circle A2 centre (-26.282, 25.0532) radius 2.975
  dimension "d48" = 5.95
  dimension "d49" = 5.95
  dimension "d50" = 4.5
  dimension "d51" = 4.5
  measures "d48" diameter of A1
  measures "d49" diameter of A2
  measures "d50" vertical distance of A0.centre A1.centre
  measures "d51" vertical distance of A0.centre A2.centre
extrude "Extrude5" cut sketch "Sketch5" against normal blind 2.93 contours A1 | A2
sketch "Sketch6" plane through (0, 3, 0) normal (0, 1, 0) x (-1, 0, 0)
  arc A0 (-46.0121, 6.1656) -> (-39.8276, 1.308) centre (-41.0121, 6.1656) ccw
  line L0 (-39.8276, 1.308) -> (-9.8276, 8.6229)
  arc A1 (-9.8276, 8.6229) -> (-6.0121, 13.4806) centre (-11.0121, 13.4806) ccw
  line L1 (-6.0121, 13.4806) -> (-6.0121, 45.6726)
  arc A2 (-6.0121, 45.6726) -> (-9.7713, 50.5162) centre (-11.0121, 45.6726) ccw
  line L2 (-9.7713, 50.5162) -> (-39.7713, 58.2013)
  arc A3 (-39.7713, 58.2013) -> (-46.0121, 53.3577) centre (-41.0121, 53.3577) ccw
  line L3 (-46.0121, 53.3577) -> (-46.0121, 6.1656)
  line L4 (-31.0121, 42.4532) -> (-31.0121, 45.4532)
  line L5 (-31.0121, 45.4532) -> (-21.0121, 45.4532)
  line L6 (-21.0121, 45.4532) -> (-21.0121, 42.4532)
  line L7 (-21.0121, 42.4532) -> (-31.0121, 42.4532)
  line L8 (-31.0121, 13.6532) -> (-31.0121, 16.6532)
  line L9 (-31.0121, 16.6532) -> (-21.0121, 16.6532)
  line L10 (-21.0121, 16.6532) -> (-21.0121, 13.6532)
  line L11 (-21.0121, 13.6532) -> (-31.0121, 13.6532)
  circle A4 centre (-26.0121, 29.5532) radius 12
  line L12 (-21.0121, 17.9232) -> (-31.0121, 17.9232)
  line L13 (-31.0121, 17.9232) -> (-31.0121, 12.3832)
  line L14 (-31.0121, 12.3832) -> (-21.0121, 12.3832)
  line L15 (-21.0121, 12.3832) -> (-21.0121, 17.9232)
  line L16 (-21.0121, 17.9232) -> (-31.0121, 12.3832) construction
  line L17 (-31.0121, 17.9232) -> (-21.0121, 12.3832) construction
  line L18 (-31.0121, 41.1832) -> (-21.0121, 41.1832)
  line L19 (-21.0121, 41.1832) -> (-21.0121, 46.7232)
  line L20 (-21.0121, 46.7232) -> (-31.0121, 46.7232)
  line L21 (-31.0121, 46.7232) -> (-31.0121, 41.1832)
  line L22 (-31.0121, 41.1832) -> (-21.0121, 46.7232) construction
  line L23 (-21.0121, 41.1832) -> (-31.0121, 46.7232) construction
  point P0 (-26.0121, 15.1532)
  point P1 (-26.0121, 43.9532)
  dimension "d52" = 10
  dimension "d53" = 5.54
  dimension "d54" = 5.54
  constraint horizontal L12
  constraint perpendicular L12 L13
  constraint parallel L12 L14
  constraint parallel L13 L15
  constraint coincident L16 P0
  constraint coincident L17 P0
  constraint horizontal L18
  constraint perpendicular L18 L19
  constraint parallel L18 L20
  constraint parallel L19 L21
  constraint coincident L22 P1
  constraint coincident L23 P1
  measures "d52" distance of L13.end L14.end
  measures "d53" distance of L12.end L13.end
  measures "d54" distance of L18.end L19.end
extrude "Extrude6" cut sketch "Sketch6" along normal blind 11 contours L7 A4 L18 L19 L21 | A4 L18 | A4 L12 | L9 A4 L12 L13 L15
equation "d12 = ( 29 / 2 ) * 1 mm"
equation "d26 = 37 mm - 10 mm - 5 mm"

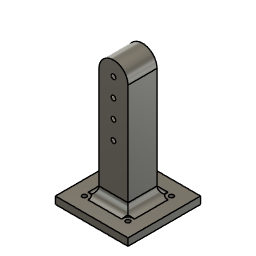
design "camera stand"
Autodesk Fusion 360 part; units mm, degrees
sketch "Sketch1" plane through (0, 0, 0) normal (0, 1, 0) x (1, 0, 0)
  line L0 (0, 0) -> (50, 0)
  line L1 (50, 0) -> (50, -50)
  line L2 (50, -50) -> (0, -50)
  line L3 (0, -50) -> (0, 0)
  dimension "d1" = 50
  dimension "d2" = 50
  constraint horizontal L0
  constraint vertical L1
  constraint horizontal L2
  constraint vertical L3
  constraint coincident L0.start L3.end
  measures "d1" distance of L0.start L0.end
  measures "d2" distance of L0.start L2.end
extrude "Extrude1" add sketch "Sketch1" along normal blind 5
sketch "Sketch2" plane through (0, 5, 0) normal (0, 1, 0) x (-1, 0, 0)
  line L0 (0, 50) -> (-50, 50)
  line L1 (-50, 50) -> (-50, 0)
  line L2 (-50, 0) -> (0, 0)
  line L3 (0, 0) -> (0, 50)
  line L4 (-35.0043, 15.0162) -> (-15.0043, 15.0162)
  line L5 (-15.0043, 15.0162) -> (-15.0043, 35.0162)
  line L6 (-15.0043, 35.0162) -> (-35.0043, 35.0162)
  line L7 (-35.0043, 35.0162) -> (-35.0043, 15.0162)
  line L8 (-35.0043, 15.0162) -> (-15.0043, 35.0162) construction
  line L9 (-15.0043, 15.0162) -> (-35.0043, 35.0162) construction
  point P0 (-25.0043, 25.0162)
  dimension "d5" = 20
  dimension "d6" = 20
  constraint horizontal L4
  constraint perpendicular L4 L5
  constraint parallel L4 L6
  constraint parallel L5 L7
  constraint coincident L8 P0
  constraint coincident L9 P0
  measures "d5" distance of L5.end L6.end
  measures "d6" distance of L4.end L5.end
extrude "Extrude2" add sketch "Sketch2" along normal blind 76.2 contours L4 L5 L6 L7
sketch "Sketch3" plane through (0, 0, 35.0162) normal (0, 0, 1) x (1, 0, 0)
  line L0 (15.0043, 5) -> (35.0043, 5)
  line L1 (35.0043, 5) -> (35.0043, 81.2)
  line L2 (35.0043, 81.2) -> (15.0043, 81.2)
  line L3 (15.0043, 81.2) -> (15.0043, 5)
  arc A0 (35.0043, 81.2) -> (15.0043, 81.2) centre (25.0043, 81.2) ccw
  constraint midpoint L2 A0.centre
extrude "Extrude3" add sketch "Sketch3" against normal blind 20 contours L2 A0
sketch "Sketch4" plane through (0, 0, 35.0162) normal (0, 0, 1) x (1, 0, 0)
  line L0 (15.0043, 5) -> (35.0043, 5)
  line L1 (35.0043, 5) -> (35.0043, 81.2)
  arc A0 (35.0043, 81.2) -> (15.0043, 81.2) centre (25.0043, 81.2) ccw
  line L2 (15.0043, 81.2) -> (15.0043, 5)
  circle A1 centre (25.0043, 81.2) radius 1.6
  dimension "d11" = 3.2
  constraint concentric A0 A1
  measures "d11" diameter of A1
extrude "Extrude4" cut sketch "Sketch4" against normal blind 70 contours A1
pattern_linear "R-Pattern1" count 4 spacing 12.7 along (0, -1, 0) of "Extrude4"
sketch "Sketch5" plane through (0, 0, 0) normal (0, -1, 0) x (1, 0, 0)
  line L0 (50, 50) -> (0, 50)
  line L1 (0, 50) -> (0, 0)
  line L2 (0, 0) -> (50, 0)
  line L3 (50, 0) -> (50, 50)
  circle A0 centre (10, 10) radius 1.5
  circle A1 centre (10, 40) radius 1.5
  circle A2 centre (40, 10) radius 1.5
  circle A3 centre (40, 40) radius 1.5
  line L4 (10, 40) -> (40, 40)
  dimension "d18" = 3
  dimension "d20" = 3
  dimension "d21" = 30
  dimension "d22" = 3
  dimension "d23" = 3
  dimension "d24" = 30
  dimension "d25" = 30
  dimension "d26" = 30
  constraint coincident A1.centre L4.start
  constraint coincident A3.centre L4.end
  measures "d18" diameter of A0
  measures "d20" diameter of A1
  measures "d21" distance of A0.centre A1.centre
  measures "d22" diameter of A2
  measures "d23" diameter of A3
  measures "d24" distance of A2.centre A3.centre
  measures "d25" distance of A0.centre A2.centre
  measures "d26" horizontal distance of A1.centre A3.centre
extrude "Extrude5" cut sketch "Sketch5" against normal blind 25 contours A0 | A1 | A2 | A3
sketch "Sketch6" plane through (0, 5, 0) normal (0, 1, 0) x (-1, 0, 0)
  circle A0 centre (-10, 10) radius 1.5
  circle A1 centre (-10, 40) radius 1.5
  circle A2 centre (-40, 10) radius 1.5
  circle A3 centre (-40, 40) radius 1.5
  line L0 (-35.0043, 35.0162) -> (-15.0043, 35.0162)
  line L1 (-15.0043, 35.0162) -> (-15.0043, 15.0162)
  line L2 (-15.0043, 15.0162) -> (-35.0043, 15.0162)
  line L3 (-35.0043, 15.0162) -> (-35.0043, 35.0162)
  line L4 (0, 50) -> (-50, 50)
  line L5 (-50, 50) -> (-50, 0)
  line L6 (-50, 0) -> (0, 0)
  line L7 (0, 0) -> (0, 50)
  circle A4 centre (-10, 40) radius 3.5
  circle A5 centre (-40, 40) radius 3.5
  circle A6 centre (-40, 10) radius 3.5
  circle A7 centre (-10, 10) radius 3.5
  dimension "d31" = 7
  dimension "d32" = 7
  dimension "d33" = 7
  dimension "d34" = 7
  constraint concentric A1 A4
  constraint concentric A3 A5
  constraint concentric A2 A6
  constraint concentric A0 A7
  measures "d31" diameter of A4
  measures "d32" diameter of A5
  measures "d33" diameter of A6
  measures "d34" diameter of A7
fillet "Fillet1" radius 6 4 edges at (25.0043, 5, 35.0162) (35.0043, 5, 25.0162) (15.0043, 5, 25.0162) (25.0043, 5, 15.0162)
extrude "Extrude6" cut sketch "Sketch6" along normal blind 5 contours A4 | A5 | A6 | A7

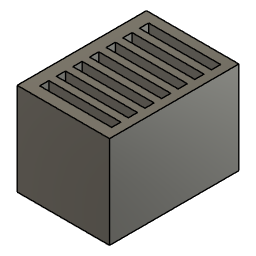
design "Jetson"
Autodesk Fusion 360 part; units mm, degrees
sketch "Sketch1" plane through (0, 0, 0) normal (0, 1, 0) x (1, 0, 0)
  line L0 (0, 0) -> (50, 0)
  line L1 (50, 0) -> (50, -70)
  line L2 (50, -70) -> (0, -70)
  line L3 (0, -70) -> (0, 0)
  constraint horizontal L0
  constraint vertical L1
  constraint horizontal L2
  constraint vertical L3
  constraint coincident L0.start L3.end
extrude "Extrude1" add sketch "Sketch1" along normal blind 50
sketch "Sketch2" plane through (0, 50, 0) normal (0, 1, 0) x (-1, 0, 0)
  line L0 (0, 70) -> (-50, 70)
  line L1 (-50, 70) -> (-50, 0)
  line L2 (-50, 0) -> (0, 0)
  line L3 (0, 0) -> (0, 70)
  line L4 (-6.3709, 5.1911) -> (-45.3042, 5.1911)
  line L5 (-45.3042, 5.1911) -> (-45.3042, 10.1463)
  line L6 (-45.3042, 10.1463) -> (-6.3709, 10.1463)
  line L7 (-6.3709, 10.1463) -> (-6.3709, 5.1911)
  line L8 (-45.3042, 14.1911) -> (-45.3042, 19.1463)
  line L9 (-45.3042, 19.1463) -> (-6.3709, 19.1463)
  line L10 (-6.3709, 14.1911) -> (-45.3042, 14.1911)
  line L11 (-6.3709, 19.1463) -> (-6.3709, 14.1911)
  line L12 (-45.3042, 23.1911) -> (-45.3042, 28.1463)
  line L13 (-45.3042, 28.1463) -> (-6.3709, 28.1463)
  line L14 (-6.3709, 23.1911) -> (-45.3042, 23.1911)
  line L15 (-6.3709, 28.1463) -> (-6.3709, 23.1911)
  line L16 (-45.3042, 32.1911) -> (-45.3042, 37.1463)
  line L17 (-45.3042, 37.1463) -> (-6.3709, 37.1463)
  line L18 (-6.3709, 32.1911) -> (-45.3042, 32.1911)
  line L19 (-6.3709, 37.1463) -> (-6.3709, 32.1911)
  line L20 (-45.3042, 41.1911) -> (-45.3042, 46.1463)
  line L21 (-45.3042, 46.1463) -> (-6.3709, 46.1463)
  line L22 (-6.3709, 41.1911) -> (-45.3042, 41.1911)
  line L23 (-6.3709, 46.1463) -> (-6.3709, 41.1911)
  line L24 (-45.3042, 50.1911) -> (-45.3042, 55.1463)
  line L25 (-45.3042, 55.1463) -> (-6.3709, 55.1463)
  line L26 (-6.3709, 50.1911) -> (-45.3042, 50.1911)
  line L27 (-6.3709, 55.1463) -> (-6.3709, 50.1911)
  line L28 (-45.3042, 59.1911) -> (-45.3042, 64.1463)
  line L29 (-45.3042, 64.1463) -> (-6.3709, 64.1463)
  line L30 (-6.3709, 59.1911) -> (-45.3042, 59.1911)
  line L31 (-6.3709, 64.1463) -> (-6.3709, 59.1911)
  dimension "d5" = 0
  dimension "d6" = 9
  constraint horizontal L4
  constraint vertical L5
  constraint horizontal L6
  constraint vertical L7
shell "Shell1" thickness 5 removed faces 1 at (16.6667, 0, 23.3333)
extrude "Extrude2" cut sketch "Sketch2" against normal blind 50 contours L4 L5 L6 L7 | L8 L9 L10 L11 | L12 L13 L14 L15 | L16 L17 L18 L19 | L20 L21 L22 L23 | L24 L25 L26 L27 | L28 L29 L30 L31
sketch "Sketch3" plane through (0, 0, 0) normal (0, -1, 0) x (1, 0, 0)
  line L0 (45.3042, 23.1911) -> (45, 23.1911)
  line L1 (45, 23.1911) -> (45, 19.1463)
  line L2 (45, 19.1463) -> (45.3042, 19.1463)
  line L3 (45.3042, 19.1463) -> (45.3042, 14.1911)
  line L4 (45.3042, 14.1911) -> (45, 14.1911)
  line L5 (45, 14.1911) -> (45, 10.1463)
  line L6 (45, 10.1463) -> (45.3042, 10.1463)
  line L7 (45.3042, 10.1463) -> (45.3042, 5.1911)
  line L8 (45.3042, 5.1911) -> (45, 5.1911)
  line L9 (45, 5.1911) -> (45, 5)
  line L10 (45, 5) -> (5, 5)
  line L11 (5, 5) -> (5, 65)
  line L12 (5, 65) -> (45, 65)
  line L13 (45, 65) -> (45, 64.1463)
  line L14 (45, 64.1463) -> (45.3042, 64.1463)
  line L15 (45.3042, 64.1463) -> (45.3042, 59.1911)
  line L16 (45.3042, 59.1911) -> (45, 59.1911)
  line L17 (45, 59.1911) -> (45, 55.1463)
  line L18 (45, 55.1463) -> (45.3042, 55.1463)
  line L19 (45.3042, 55.1463) -> (45.3042, 50.1911)
  line L20 (45.3042, 50.1911) -> (45, 50.1911)
  line L21 (45, 50.1911) -> (45, 46.1463)
  line L22 (45, 46.1463) -> (45.3042, 46.1463)
  line L23 (45.3042, 46.1463) -> (45.3042, 41.1911)
  line L24 (45.3042, 41.1911) -> (45, 41.1911)
  line L25 (45, 41.1911) -> (45, 37.1463)
  line L26 (45, 37.1463) -> (45.3042, 37.1463)
  line L27 (45.3042, 37.1463) -> (45.3042, 32.1911)
  line L28 (45.3042, 32.1911) -> (45, 32.1911)
  line L29 (45, 32.1911) -> (45, 28.1463)
  line L30 (45, 28.1463) -> (45.3042, 28.1463)
  line L31 (45.3042, 28.1463) -> (45.3042, 23.1911)
  line L32 (50, 70) -> (0, 70)
  line L33 (0, 70) -> (0, 0)
  line L34 (0, 0) -> (50, 0)
  line L35 (50, 0) -> (50, 70)
  line L36 (50, 0) -> (0, 0)
  line L37 (0, 0) -> (0, 70)
  line L38 (0, 70) -> (50, 70)
  line L39 (50, 70) -> (50, 0)
  constraint horizontal L36
  constraint vertical L37
  constraint horizontal L38
  constraint vertical L39
  constraint coincident L32.end L33.start
  constraint coincident L34.end L35.start
extrude "Extrude3" add sketch "Sketch3" against normal blind 5 contours L0 L1 L2 L3 L4 L5 L6 L7 L8 L9 L10 L11 L12 L13 L14 L15 L16 L17 L18 L19 L20 L21 L22 L23 L24 L25 L26 L27 L28 L29 L30 L31

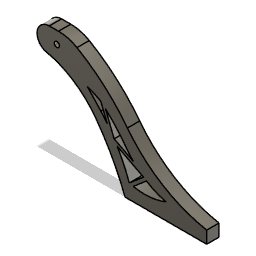
design "Hinge arm"
Autodesk Fusion 360 part; units mm, degrees
sketch "Sketch1" plane through (0, 0, 0) normal (0, 0, 1) x (1, 0, 0)
  line L0 (0, 0) -> (50, 0)
  line L1 (50, 0) -> (50, 7.5)
  line L2 (50, 7.5) -> (27.9792, 7.5)
  line L3 (-46.3191, 63.75) -> (-46.3191, 56.25)
  circle A0 centre (-41.6596, 60) radius 1.6
  line L4 (50, 7.5) -> (17.5, 7.5)
  line L5 (-46.3191, 60) -> (-46.3191, 67.5)
  line L6 (-46.3191, 60) -> (-46.3191, 52.5)
  line L7 (-46.3191, 67.5) -> (-35, 67.5)
  line L8 (-46.3191, 52.5) -> (-35.3669, 52.5)
  arc A1 (17.5, 7.5) -> (-35, 67.5) centre (-82.3864, -26.9318) ccw
  arc A2 (0, 0) -> (-35.3669, 52.5) centre (-129.8244, -49.2943) ccw
  dimension "d1" = 50
  dimension "d29" = 3.2
  dimension "d42" = 22.0208
  dimension "d43" = 32.5
  dimension "d50" = 7.5
  dimension "d51" = 7.5
  constraint horizontal L0
  constraint vertical L1
  constraint coincident L0.start A2.start
  constraint vertical L3
  constraint perpendicular L1 L4
  constraint midpoint L3 L5.start
  constraint parallel L3 L5
  constraint parallel L3 L6
  constraint perpendicular L5 L7
  constraint perpendicular L6 L8
  measures "d1" distance of L0.start L0.end
  measures "d29" diameter of A0
  measures "d42" distance of L1.end L2.end
  measures "d43" distance of L1.end L4.end
  measures "d50" distance of L5.start L5.end
  measures "d51" distance of L5.start L6.end
extrude "Extrude1" add sketch "Sketch1" along normal blind 7.5
sketch "Sketch3" plane through (0, 0, 0) normal (0, -1, 0) x (1, 0, 0)
  line L0 (0, 0) -> (50, 0)
  line L1 (50, 0) -> (50, 7.5)
  line L2 (50, 7.5) -> (0, 7.5)
  circle A0 centre (10, 3.75) radius 2.45
  circle A1 centre (25, 3.75) radius 2.45
  circle A2 centre (40, 3.75) radius 2.45
  line L3 (0, 7.5) -> (0, 0)
  dimension "d21" = 4.9
  dimension "d23" = 4.9
  dimension "d24" = 15
  dimension "d25" = 4.9
  dimension "d26" = 15
  measures "d21" diameter of A0
  measures "d23" diameter of A1
  measures "d24" distance of A0.centre A1.centre
  measures "d25" diameter of A2
  measures "d26" distance of A1.centre A2.centre
fillet "Fillet11" radius 79.5 1 edges at (17.5, 7.5, 3.75)
fillet "Fillet12" radius 22.5 1 edges at (-35, 67.5, 3.75)
fillet "Fillet13" radius 52.5 1 edges at (-35.3669, 52.5, 3.75)
extrude "Extrude3" cut sketch "Sketch3" against normal blind 5 contours A0 | A1 | A2